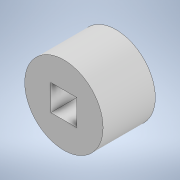
# Autodesk Inventor part: ArmCylinder
Saved by Autodesk Inventor 2021 (Build 250183000, 183)
## iProperties
Created: 2024-05-10
Part Number: ArmCylinder
Material: Generic
Document SubType Name: Modeling
Designer: brybr
Density: 1 g/cm^3
Appearance: Default
Author: brybr
Autodesk Inventor part; units mm, degrees
ref_plane "YZ Plane" through (0, 0, 0) normal (1, 0, 0) x (0, 1, 0)
ref_plane "XZ Plane" through (0, 0, 0) normal (0, 1, 0) x (-1, 0, 0)
ref_plane "XY Plane" through (0, 0, 0) normal (0, 0, 1) x (1, 0, 0)
sketch "Sketch1" plane through (0, 0, 0) normal (0, 0, 1) x (1, 0, 0)
  circle A0 centre (0, 0) radius 7.5
  line L0 (2.5, -2.5) -> (-2.5, -2.5)
  line L1 (-2.5, -2.5) -> (-2.5, 2.5)
  line L2 (-2.5, 2.5) -> (2.5, 2.5)
  line L3 (2.5, 2.5) -> (2.5, -2.5)
  line L4 (2.5, -2.5) -> (-2.5, 2.5) construction
  line L5 (-2.5, -2.5) -> (2.5, 2.5) construction
  dimension "d0" = 15
  dimension "d1" = 5
  dimension "d2" = 5
  constraints: 12 end point, 2 midpoint, 2 parallel, 1 centre point, 1 coincident, 1 horizontal, 1 perpendicular
  measures "d0" diameter of A0
  measures "d1" distance of L1.end L2.end
  measures "d2" distance of L0.end L1.end
extrude "Extrusion1" add sketch "Sketch1" along normal blind 10
body "Solid1"
